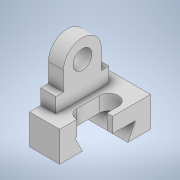
# Autodesk Inventor part: Урок
Saved by Autodesk Inventor 2022 (Build 260153000, 153)
## iProperties
Created: 2023-04-14
Part Number: Урок
Material: Типовые
Document SubType Name: Modeling
Designer: Egor
Density: 1 g/cm^3
Appearance: По умолчанию
Author: Egor
Autodesk Inventor part; units mm, degrees
ref_plane "YZ Plane" through (0, 0, 0) normal (1, 0, 0) x (0, 1, 0)
ref_plane "XZ Plane" through (0, 0, 0) normal (0, 1, 0) x (-1, 0, 0)
sketch "Эскиз1" plane through (0, 0, 0) normal (0, 1, 0) x (-1, 0, 0)
  line L0 (30, 50) -> (30, -50)
  line L1 (30, -50) -> (-30, -50)
  line L2 (-30, -50) -> (-30, 50)
  line L3 (-30, 50) -> (30, 50)
  point P0 (0, 0)
  dimension "d2" = 100
  dimension "d3" = 60
  dimension "d4" = 100
  constraints: 8 end point, 1 perpendicular
  measures "d2" distance of L0.start L0.end
  measures "d3" distance of L0.end L1.end
  measures "d4" distance of L1.end L2.end
extrude "Выдавливание1" add sketch "Эскиз1" along normal blind 40
sketch "Эскиз2" plane through (30, 0, 50) normal (1, 0, 0) x (0, 0, -1)
  line L0 (30, 0) -> (70, 0)
  line L1 (20, 20) -> (80, 20)
  line L2 (80, 20) -> (70, 0)
  line L3 (20, 20) -> (30, 0)
  point P0 (50, 0)
  dimension "d8" = 40
  dimension "d11" = 60
  constraints: 8 end point
  measures "d8" distance of L0.start L0.end
  measures "d11" distance of L1.start L1.end
extrude "Выдавливание2" cut sketch "Эскиз2" along normal mid plane 160
sketch "Эскиз4" plane through (0, 40, 0) normal (0, 1, 0) x (1, 0, 0)
  line L0 (30, -30) -> (30, 30) projected
  line L1 (30, -50) -> (30, 50) projected
  arc A0 (22.5, 15) -> (-2.5, 15) centre (10, 15) ccw
  arc A1 (-2.5, -15) -> (22.5, -15) centre (10, -15) ccw
  line L2 (-2.5, 15) -> (-2.5, -15)
  line L3 (22.5, 15) -> (22.5, -15)
  point P0 (0, 0)
  constraints: 4 end point, 4 point on circle, 2 centre point, 1 parallel, 1 tangent
extrude "Выдавливание5" cut sketch "Эскиз4" against normal blind 20
sketch "Эскиз5" plane through (-30, 0, 50) normal (-1, 0, 0) x (0, 0, 1)
  line L0 (0, 40) -> (-100, 40) projected
  line L1 (-100, 40) -> (-85, 40)
  line L2 (-85, 40) -> (-15, 40)
  line L3 (-85, 40) -> (-85, 60)
  line L4 (-85, 60) -> (-75, 60)
  line L5 (-15, 40) -> (-15, 60)
  line L6 (-15, 60) -> (-25, 60)
  line L7 (-25, 60) -> (-25, 85)
  line L8 (-75, 60) -> (-75, 85)
  arc A0 (-25, 85) -> (-75, 85) centre (-50, 85) ccw
  line L9 (-75, 85) -> (-25, 85)
  circle A1 centre (-50, 85) radius 12.5
  point P0 (-50, 0)
  dimension "d50" = 70
  dimension "d51" = 20
  dimension "d52" = 10
  dimension "d53" = 20
  dimension "d54" = 10
  dimension "d55" = 25
  dimension "d56" = 25
  dimension "d59" = 25
  constraints: 18 end point, 4 perpendicular, 2 centre point, 2 point on circle, 2 point on line, 2 vertical, 1 coincident
  measures "d50" distance of L1.end L2.end
  measures "d51" distance of L1.end L3.end
  measures "d52" distance of L3.end L4.end
  measures "d53" distance of L2.end L5.end
  measures "d54" distance of L5.end L6.end
  measures "d55" distance of L6.end L7.end
  measures "d56" distance of L4.end L8.end
  measures "d59" diameter of A1
extrude "Выдавливание6" add sketch "Эскиз5" against normal blind 20 contours L0 L3 L4 L8 L9 A1 L7 L6 L5 | L9 A1 A0
ref_plane "РабПлоскость1" through (10, 0, -50) normal (1, 0, 0) x (0, 0, -1)
sketch "Эскиз6" plane through (0, 40, 0) normal (0, 1, 0) x (1, 0, 0)
  arc A0 (-2.5, -15) -> (22.5, -15) centre (10, -15) ccw projected
  line L0 (10, -15) -> (10, -69.4027)
  line L1 (10, -69.4027) -> (54.89, -69.4027)
  line L2 (54.89, -69.4027) -> (54.89, -15)
  line L3 (10, -15) -> (10, 0)
  line L4 (10, 0) -> (54.89, 0)
  line L5 (54.89, 0) -> (54.89, -15)
  point P0 (0, 0)
  dimension "d65" = 12.5
  constraints: 12 end point, 4 perpendicular, 1 vertical
  measures "d65" distance of A0.end L0.start
extrude "Выдавливание7" cut sketch "Эскиз6" against normal blind 80
